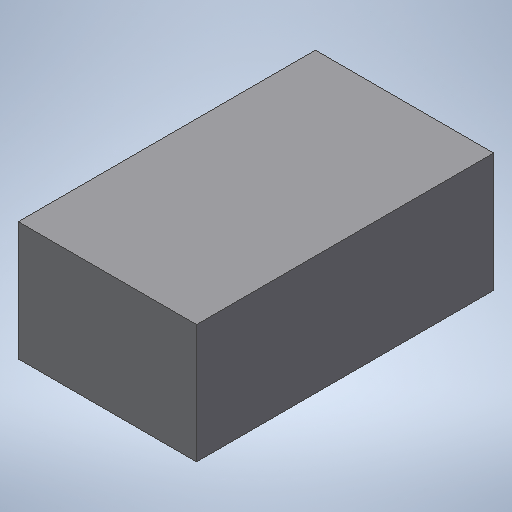
# Autodesk Inventor part: SamplePart
Saved by Autodesk Inventor 2027 (Build 310192060, 192F)
## iProperties
Created: 2026-06-17
Part Number: SamplePart
Material: Generisch
Document SubType Name: Modeling
Designer: tobia
Density: 1 g/cm^3
Appearance: Vorgabe
Project: Proj1
DateTest: 2026-06-17
Author: tobia
ThisIsATest: Primary
SecondProp: Primary
BoolTest: False
NumberTest: 0
Title: Test1
Autodesk Inventor part; units mm, degrees
ref_plane "YZ Plane" through (0, 0, 0) normal (1, 0, 0) x (0, 1, 0)
ref_plane "XZ Plane" through (0, 0, 0) normal (0, 1, 0) x (-1, 0, 0)
ref_plane "XY Plane" through (0, 0, 0) normal (0, 0, 1) x (1, 0, 0)
sketch "Sketch1" plane through (0, 0, 0) normal (0, 1, 0) x (-1, 0, 0)
  line L0 (-7.5, -12.5) -> (7.5, -12.5)
  line L1 (7.5, -12.5) -> (7.5, 12.5)
  line L2 (7.5, 12.5) -> (-7.5, 12.5)
  line L3 (-7.5, 12.5) -> (-7.5, -12.5)
  line L4 (-7.5, -12.5) -> (7.5, 12.5) construction
  line L5 (7.5, -12.5) -> (-7.5, 12.5) construction
  point P0 (0, 0)
  dimension "d0" = 15
  dimension "d1" = 25
  constraints: 12 end point, 2 midpoint, 2 parallel, 1 horizontal, 1 perpendicular
  measures "d0" distance of L2.end L1.end
  measures "d1" distance of L1.end L0.end
extrude "Extrusion1" add sketch "Sketch1" along normal blind 10
chamfer "Chamfer1" [suppressed]
sketch "Sketch3" plane through (0, 10, 0) normal (0, 1, 0) x (1, 0, 0)
  point P0 (0, 0)
  point P1 (0.0394, 0.1841)
feature "Slot1" [suppressed]
body "Solid1"
